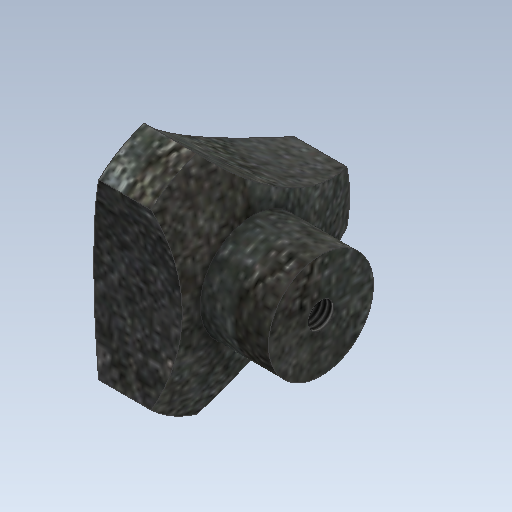
# Autodesk Inventor part: fogantyu
Saved by Autodesk Inventor 2021.4 (Build 254397000, 397)
## iProperties
Created: 2023-12-02
Part Number: fogantyu
Material: Steel
Document SubType Name: Modeling
Designer: vtoth
Density: 7.85 g/cm^3
Appearance: Plate
Mass: 146.973 g
Surface Area: 49.6309 cm^2
Volume: 18.7227 cm^3
Author: vtoth
Autodesk Inventor part; units mm, degrees
ref_plane "YZ Plane" through (0, 0, 0) normal (1, 0, 0) x (0, 1, 0)
ref_plane "XZ Plane" through (0, 0, 0) normal (0, 1, 0) x (-1, 0, 0)
ref_plane "XY Plane" through (0, 0, 0) normal (0, 0, 1) x (1, 0, 0)
sketch "Sketch1" plane through (0, 0, 0) normal (0, 0, 1) x (1, 0, 0)
  line L0 (0, 27.3257) -> (0, -4.5543) construction
  line L1 (-50.8151, 0) -> (70.7599, 0) construction
  line L2 (32, 0) -> (32, 10)
  line L3 (32, 10) -> (19, 10)
  line L4 (14.9724, 22.5) -> (4.9724, 22.5)
  arc A0 (4.9724, 22.5) -> (0, 0) centre (53.3921, 0) ccw
  arc A1 (19.9448, 0) -> (14.9724, 22.5) centre (-33.4472, 0) ccw
  line L5 (9.9724, 22.5) -> (9.9724, 17.1499) construction
  line L6 (32, 0) -> (0, 0)
  dimension "d0" = 20
  dimension "d1" = 45
  dimension "d2" = 32
  dimension "d3" = 10
  dimension "d4" = 13
  constraints: 10 end point, 6 point on circle, 3 point on line, 2 centre point, 2 perpendicular, 2 vertical, 1 line through centre, 1 midpoint, 1 parallel, 1 other
  measures "d0" diameter of L3 L1
  measures "d1" diameter of L4 L1
  measures "d2" distance edge to line of A0 L2
  measures "d3" distance of L4.end L4.start
  measures "d4" distance of L3.end L2.end
revolve "Revolution1" add sketch "Sketch1" angle 360 about axis through (0, 0, 0) along (1, 0, 0)
sketch "Sketch2" plane through (0, 0, 0) normal (1, 0, 0) x (0, 1, 0)
  circle A0 centre (0, 0) radius 22.5 construction
  line L0 (0, 31.5) -> (0, -31.5) construction
  circle A1 centre (0, 68.488) radius 55.6891
  circle A2 centre (-59.3123, -34.244) radius 55.6891
  circle A3 centre (59.3123, -34.244) radius 55.6891
  point P0 (-16.4984, 15.2988)
  point P1 (-21.4984, 6.6386)
  point P2 (0, 12.7988)
  dimension "d8" = 360
  dimension "d10" = 10
  dimension "d11" = 2.5
  constraints: 4 point on circle, 2 centre point, 2 point on line, 10 other
  measures "d10" distance of A0.start A0.end
  measures "d11" vertical distance of A0.start A1.end
extrude "Extrusion1" cut sketch "Sketch2" along normal through all
sketch "Sketch3" plane through (32, 0, 0) normal (1, 0, 0) x (0, 0, -1)
  circle A0 centre (0, 0) radius 10 projected
hole "Hole1" at (32, 0, 0) direction (-1, 0, 0) diameter 4.917 end through all thread size "M6x1" class "6H" standard "ISO Metric profile"
body "Solid1"
